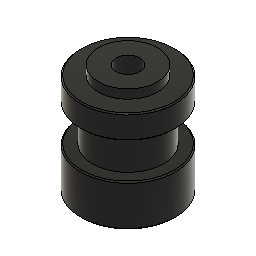
V0CableGland (Autodesk Fusion 360 archive; units mm, degrees)
design "Dragon Groovemount"
Autodesk Fusion 360 part; units mm, degrees
sketch "Sketch1" plane through (0, 0, 0) normal (0, 0, 1) x (1, 0, 0)
  line L0 (0, 0) -> (0, 70.4213)
  line L1 (0, 0) -> (8, 0)
  line L2 (8, 0) -> (8, 7)
  line L3 (8, 7) -> (6, 7)
  line L4 (6, 7) -> (6, 13)
  line L5 (6, 13) -> (8, 13)
  line L6 (8, 13) -> (8, 17)
  line L7 (8, 17) -> (0, 17)
  line L8 (2, 18.5) -> (2, 0)
  line L9 (5, 17) -> (5, 18.5)
  line L10 (5, 18.5) -> (0, 18.5)
  dimension "d1" = 17
  dimension "d2" = 4
  dimension "d3" = 7
  dimension "d4" = 12
  dimension "d5" = 16
  dimension "d6" = 1.5
  dimension "d7" = 10
  dimension "d8" = 4
  constraint coincident L0.start L1.start
  constraint vertical L0
  constraint perpendicular L0 L1
  constraint perpendicular L1 L2
  constraint perpendicular L2 L3
  constraint perpendicular L1 L4
  constraint perpendicular L2 L5
  constraint perpendicular L5 L6
  constraint coincident L0 L7.end
  constraint perpendicular L0 L7
  constraint collinear L2 L6
  constraint coincident L1 L8.end
  constraint perpendicular L1 L8
  constraint coincident L7 L9.start
  constraint perpendicular L7 L9
  constraint coincident L0 L10.end
  constraint perpendicular L0 L10
  constraint coincident L10 L8.start
  measures "d1" distance of L1 L7
  measures "d2" distance of L5.end L6.end
  measures "d3" distance of L1.end L2.end
  measures "d6" distance of L9.start L9.end
revolve "Revolve1" add sketch "Sketch1" angle 360 about axis through (0, 0, 0) along (0, 1, 0) contours L1 L2 L3 L4 L5 L6 L7 L8 | L7 L8 L9 L10
sketch "Sketch2" plane through (0, 0, 0) normal (0, 1, 0) x (1, 0, 0)
  line L0 (0, 0) -> (6, 0) construction
  line L1 (0, 0) -> (-6, 0) construction
  circle A0 centre (-6, 0) radius 1
  circle A1 centre (6, 0) radius 1
  dimension "d10" = 2
  dimension "d11" = 6
  constraint coincident L0.start L1.start
  constraint horizontal L0
  constraint parallel L0 L1
  constraint equal L0 L1
  constraint coincident L1.end A0.centre
  constraint coincident L0.end A1.centre
  constraint equal A0 A1
  measures "d10" diameter of A0
  measures "d11" distance of L0.start L1.end
extrude "Extrude1" cut sketch "Sketch2" along normal blind 5
chamfer "Chamfer1" distance 0.2 angle 45 4 edges at (-7.4586, 17, -2.8929) (-7.4586, 7, -2.8929) (-7.4586, 13, -2.8929) (-7.4586, 0, -2.8929)
